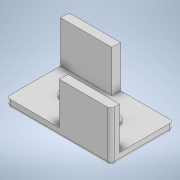
# Autodesk Inventor part: 2Wide5mm
Saved by Autodesk Inventor 2022 (Build 260153000, 153)
## iProperties
Created: 2020-10-30
Part Number: 2Wide5mm
Material: Generic
Document SubType Name: Modeling
Designer: PAB
Density: 1 g/cm^3
Appearance: Default
Author: PAB
Autodesk Inventor part; units mm, degrees
ref_plane "YZ Plane" through (0, 0, 0) normal (1, 0, 0) x (0, 1, 0)
ref_plane "XZ Plane" through (0, 0, 0) normal (0, 1, 0) x (-1, 0, 0)
ref_plane "XY Plane" through (0, 0, 0) normal (0, 0, 1) x (1, 0, 0)
sketch "Sketch1" plane through (0, 0, 0) normal (0, 1, 0) x (-1, 0, 0)
  line L0 (30.4, 18.2) -> (-30.4, 18.2)
  line L1 (-30.4, 18.2) -> (-30.4, -18.2)
  line L2 (-30.4, -18.2) -> (30.4, -18.2)
  line L3 (30.4, -18.2) -> (30.4, 18.2)
  point P0 (0, 0)
  dimension "d0" = 60.8
  dimension "d1" = 36.4
  constraints: 8 end point, 2 parallel, 1 horizontal, 1 perpendicular
  measures "d0" distance of L2.end L1.end
  measures "d1" distance of L1.end L0.end
extrude "Extrusion1" add sketch "Sketch1" along normal blind 5
sketch "Sketch2" plane through (0, 5, 0) normal (0, 1, 0) x (1, 0, 0)
  line L0 (30.4, 18.2) -> (-30.4, 18.2) projected
  line L1 (-30.4, 18.2) -> (-0.4, 18.2)
  line L2 (-0.4, 18.2) -> (-0.4, 13.2)
  line L3 (-0.4, 13.2) -> (-30.4, 13.2)
  line L4 (-30.4, 13.2) -> (-30.4, 18.2)
  line L5 (30.4, -18.2) -> (30.4, 18.2) projected
  line L6 (30.4, -18.2) -> (0.4, -18.2)
  line L7 (0.4, -18.2) -> (0.4, -13.2)
  line L8 (0.4, -13.2) -> (30.4, -13.2)
  line L9 (30.4, -13.2) -> (30.4, -18.2)
  point P0 (0, 0)
  dimension "d4" = 30
  dimension "d5" = 5
  dimension "d6" = 30
  dimension "d7" = 5
  constraints: 16 end point, 4 parallel, 2 horizontal, 2 perpendicular
  measures "d4" distance of L2.end L3.end
  measures "d5" distance of L1.end L2.end
  measures "d6" distance of L7.end L8.end
  measures "d7" distance of L6.end L7.end
extrude "Extrusion2" add sketch "Sketch2" along normal blind 24.4
sketch "Sketch3" plane through (0, 5, 0) normal (0, 1, 0) x (1, 0, 0)
  circle A0 centre (12.7, 0) radius 4.325
  circle A1 centre (-12.7, 0) radius 4.325
  point P0 (0, 0)
  dimension "d10" = 8.65
  dimension "d11" = 8.65
  constraints: 2 centre point
  measures "d10" diameter of A0
  measures "d11" diameter of A1
extrude "Extrusion3" add sketch "Sketch3" along normal blind 3
sketch "Sketch4" plane through (-12.7, 8, 0) normal (0, 1, 0) x (1, 0, 0)
  circle A0 centre (0, 0) radius 2
  circle A1 centre (25.4, 0) radius 4.325 projected
  circle A2 centre (25.4, 0) radius 2
  point P0 (12.7, 0)
  dimension "d14" = 4
  dimension "d15" = 4
  constraints: 2 centre point, 1 coincident
  measures "d14" diameter of A0
  measures "d15" diameter of A2
extrude "Extrusion4" cut sketch "Sketch4" against normal blind 15 contours A0 | A2
sketch "Sketch5" plane through (0, 0, 0) normal (0, -1, 0) x (1, 0, 0)
  circle A0 centre (12.7, 0) radius 2 projected
  circle A1 centre (12.7, 0) radius 3
  circle A2 centre (-12.7, 0) radius 2 projected
  circle A3 centre (-12.7, 0) radius 3
  point P0 (0, 0)
  dimension "d18" = 6
  dimension "d19" = 6
  constraints: 2 centre point, 2 coincident
  measures "d18" diameter of A1
  measures "d19" diameter of A3
extrude "Extrusion5" cut sketch "Sketch5" against normal blind 3 contours A0 | A1 | A2 | A3
chamfer "Chamfer1" distance 1.5 angle 45 2 edges at (8.375, 8, 0) (-17.025, 8, 0)
fillet "Fillet1" radius 2 8 edges at (0, 0, 18.2) (-30.4, 0, 0) (0, 0, -18.2) (30.4, 0, 0) (-30.4, 14.7, -18.2) (-30.4, 2.5, 18.2) (30.4, 14.7, 18.2) (30.4, 2.5, -18.2)
body "Solid1"
